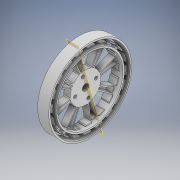
# Autodesk Inventor part: Kotač_v.3.0
Saved by Autodesk Inventor 2020 (Build 240168000, 168)
## iProperties
Created: 2020-10-18
Part Number: Kotač_v.3.0
Material: Generic
Document SubType Name: Modeling
Designer: Sičaja
Density: 1 g/cm^3
Appearance: Default
Author: Sičaja
Autodesk Inventor part; units mm, degrees
ref_plane "YZ Plane" through (0, 0, 0) normal (1, 0, 0) x (0, 1, 0)
ref_plane "XZ Plane" through (0, 0, 0) normal (0, 1, 0) x (-1, 0, 0)
ref_plane "XY Plane" through (0, 0, 0) normal (0, 0, 1) x (1, 0, 0)
sketch "Sketch1" plane through (0, 0, 0) normal (1, 0, 0) x (0, 1, 0)
  circle A0 centre (0, 0) radius 25
  dimension "d0" = 50
  constraints: 1 centre point, 1 coincident
  measures "d0" diameter of A0
extrude "Extrusion1" add sketch "Sketch1" along normal blind 7
sketch "Sketch3" plane through (7, 0, 0) normal (1, 0, 0) x (0, 0, -1)
  arc A0 (-3.1611, 20.2548) -> (-7.5525, 19.0581) centre (0, 0) ccw
  line L0 (-3.1611, 20.2548) -> (-1.4649, 9.3864)
  line L1 (-3.4999, 8.8318) -> (-7.5525, 19.0581)
  line L2 (-2.081, 9.2902) -> (-3.6795, 19.5329)
  arc A1 (-3.6795, 19.5329) -> (-6.7395, 18.699) centre (0, 0) ccw
  line L3 (-6.7395, 18.699) -> (-2.9203, 9.0615)
  circle A2 centre (0, 0) radius 9.5591
  line L4 (-17.9878, 8.4566) -> (-8.4724, 4.3425)
  line L5 (-8.7198, 3.7702) -> (-18.8165, 8.1357)
  arc A3 (-16.4137, 11.2101) -> (-17.9878, 8.4566) centre (0, 0) ccw
  arc A4 (-16.5575, 12.0871) -> (-18.8165, 8.1357) centre (0, 0) ccw
  line L6 (-16.5575, 12.0871) -> (-7.673, 5.6013)
  line L7 (-8.0406, 5.0977) -> (-16.4137, 11.2101)
  circle A5 centre (0, 0) radius 9.5591
  line L8 (-18.699, -6.7395) -> (-9.0615, -2.9203)
  line L9 (-8.8318, -3.4999) -> (-19.0581, -7.5525)
  arc A6 (-19.5329, -3.6795) -> (-18.699, -6.7395) centre (0, 0) ccw
  arc A7 (-20.2548, -3.1611) -> (-19.0581, -7.5525) centre (0, 0) ccw
  line L10 (-20.2548, -3.1611) -> (-9.3864, -1.4649)
  line L11 (-9.2902, -2.081) -> (-19.5329, -3.6795)
  circle A8 centre (0, 0) radius 9.5591
  line L12 (-8.4566, -17.9878) -> (-4.3425, -8.4724)
  line L13 (-3.7702, -8.7198) -> (-8.1357, -18.8165)
  arc A9 (-11.2101, -16.4137) -> (-8.4566, -17.9878) centre (0, 0) ccw
  arc A10 (-12.0871, -16.5575) -> (-8.1357, -18.8165) centre (0, 0) ccw
  line L14 (-12.0871, -16.5575) -> (-5.6013, -7.673)
  line L15 (-5.0977, -8.0406) -> (-11.2101, -16.4137)
  circle A11 centre (0, 0) radius 9.5591
  line L16 (6.7395, -18.699) -> (2.9203, -9.0615)
  line L17 (3.4999, -8.8318) -> (7.5525, -19.0581)
  arc A12 (3.6795, -19.5329) -> (6.7395, -18.699) centre (0, 0) ccw
  arc A13 (3.1611, -20.2548) -> (7.5525, -19.0581) centre (0, 0) ccw
  line L18 (3.1611, -20.2548) -> (1.4649, -9.3864)
  line L19 (2.081, -9.2902) -> (3.6795, -19.5329)
  circle A14 centre (0, 0) radius 9.5591
  line L20 (17.9878, -8.4566) -> (8.4724, -4.3425)
  line L21 (8.7198, -3.7702) -> (18.8165, -8.1357)
  arc A15 (16.4137, -11.2101) -> (17.9878, -8.4566) centre (0, 0) ccw
  arc A16 (16.5575, -12.0871) -> (18.8165, -8.1357) centre (0, 0) ccw
  line L22 (16.5575, -12.0871) -> (7.673, -5.6013)
  line L23 (8.0406, -5.0977) -> (16.4137, -11.2101)
  circle A17 centre (0, 0) radius 9.5591
  line L24 (18.699, 6.7395) -> (9.0615, 2.9203)
  line L25 (8.8318, 3.4999) -> (19.0581, 7.5525)
  arc A18 (19.5329, 3.6795) -> (18.699, 6.7395) centre (0, 0) ccw
  arc A19 (20.2548, 3.1611) -> (19.0581, 7.5525) centre (0, 0) ccw
  line L26 (20.2548, 3.1611) -> (9.3864, 1.4649)
  line L27 (9.2902, 2.081) -> (19.5329, 3.6795)
  circle A20 centre (0, 0) radius 9.5591
  line L28 (8.4566, 17.9878) -> (4.3425, 8.4724)
  line L29 (3.7702, 8.7198) -> (8.1357, 18.8165)
  arc A21 (11.2101, 16.4137) -> (8.4566, 17.9878) centre (0, 0) ccw
  arc A22 (12.0871, 16.5575) -> (8.1357, 18.8165) centre (0, 0) ccw
  line L30 (12.0871, 16.5575) -> (5.6013, 7.673)
  line L31 (5.0977, 8.0406) -> (11.2101, 16.4137)
  circle A23 centre (0, 0) radius 9.5591
  circle A24 centre (0, 0) radius 2 projected
  circle A25 centre (0, 0) radius 20.5
  circle A26 centre (0, 0) radius 9.5204
  point P0 (-8.5079, 4.3579)
  point P1 (-8.0719, 5.1206)
  point P2 (-9.4448, -1.474)
  point P3 (-8.7741, 3.7936)
  point P4 (-9.0975, -2.9345)
  point P5 (-9.3285, -2.0869)
  point P6 (-4.3579, -8.5079)
  point P7 (-5.1206, -8.0719)
  point P8 (-12.0871, -16.5575)
  point P9 (-5.6362, -7.7207)
  point P10 (-8.8867, -3.5217)
  point P11 (1.474, -9.4448)
  point P12 (-3.7936, -8.7741)
  point P13 (2.9345, -9.0975)
  point P14 (2.0869, -9.3285)
  point P15 (7.7207, -5.6362)
  point P16 (3.5217, -8.8867)
  point P17 (8.5079, -4.3579)
  point P18 (8.0719, -5.1206)
  point P19 (9.4448, 1.474)
  point P20 (8.7741, -3.7936)
  point P21 (9.0975, 2.9345)
  point P22 (9.3285, 2.0869)
  point P23 (19.0581, 7.5525)
  point P24 (5.6362, 7.7207)
  point P25 (8.8867, 3.5217)
  point P26 (4.3579, 8.5079)
  point P27 (5.1206, 8.0719)
  point P28 (-2.9345, 9.0975)
  point P29 (-2.0869, 9.3285)
  point P30 (-1.474, 9.4448)
  point P31 (3.7936, 8.7741)
  point P32 (-7.5525, 19.0581)
  point P33 (-16.5575, 12.0871)
  point P34 (-7.7207, 5.6362)
  point P35 (-3.5217, 8.8867)
  dimension "d15" = 41
  dimension "d18" = 360
  constraints: 64 end point, 32 point on circle, 24 centre point, 10 coincident, 2 coincident with centre, 142 other
  measures "d15" diameter of A0
extrude "Extrusion3" cut sketch "Sketch3" against normal blind 7 contours A25 L29 A2 L0 | L1 A2 L6 A25 | A2 L3 A1 L2 | A25 L25 A2 L30 | L5 A2 L10 A25 | L28 A21 L31 A2 | A2 L4 A3 L7 | A25 L21 A2 L26 | L9 A2 L14 A25 | L24 A18 L27 A2 | A2 L8 A6 L11 | L13 A2 L18 A25 | A25 L17 A2 L22 | A2 L12 A9 L15 | L20 A15 L23 A2 | A2 L16 A12 L19
sketch "Sketch4" plane through (7, 0, 0) normal (1, 0, 0) x (0, 0, -1)
  circle A0 centre (0, 0) radius 9.5
  circle A1 centre (0, 0) radius 7.8
  circle A2 centre (0, 0) radius 6.8
  circle A3 centre (0, 0) radius 2
  circle A4 centre (-1.787, 6.561) radius 1
  circle A5 centre (-6.561, -1.787) radius 1
  circle A6 centre (1.787, -6.561) radius 1
  circle A7 centre (6.561, 1.787) radius 1
  dimension "d24" = 13.6
  dimension "d22" = 19
  dimension "d23" = 15.6
  dimension "d25" = 4
  dimension "d26" = 2
  dimension "d29" = 360
  constraints: 7 centre point, 4 coincident, 12 other
  measures "d22" diameter of A0
  measures "d23" diameter of A1
  measures "d25" diameter of A3
  measures "d26" diameter of A4
extrude "Extrusion4" cut sketch "Sketch4" against normal blind 7 contours A7 A2 | A6 A2 | A4 A2 | A2 A7 | A5 A2 | A6 A2 | A4 A2 | A5 A2 | A3
sketch "Sketch5" plane through (7, 0, 0) normal (1, 0, 0) x (0, 0, -1)
  circle A0 centre (0, 0) radius 21.5
  circle A1 centre (0, 0) radius 25 projected
  circle A2 centre (0, 0) radius 23.5
  circle A3 centre (0, 0) radius 26
  dimension "d33" = 43
  dimension "d34" = 47
  dimension "d35" = 52
  constraints: 3 centre point, 3 coincident
  measures "d33" diameter of A0
  measures "d34" diameter of A2
  measures "d35" diameter of A3
extrude "Extrusion5" cut sketch "Sketch5" against normal blind 7 contours A1 | A2 | A3
ref_plane "Work Plane2" through (0, 0, 0) normal (0, -0.2629324, 0.9648142) x (-1, 0, 0)
sketch "Sketch8" plane through (0, 0, 0) normal (-1, 0, 0) x (0, 0, 1)
  circle A0 centre (0, 0) radius 2 projected
  line L0 (-0.9032, 19.8559) -> (-0.9315, 20.4788)
  line L1 (10.8505, 16.6535) -> (11.1909, 17.176)
  line L2 (5.2251, 19.1774) -> (5.6518, 20.7438)
  line L3 (2.0869, 9.3285) -> (3.6795, 19.5329) projected
  line L4 (3.1611, 20.2548) -> (1.474, 9.4448) projected
  line L5 (3.5217, 8.8867) -> (7.5525, 19.0581) projected
  line L6 (7.5525, 19.0581) -> (3.5217, 8.8867) projected
  line L7 (3.5217, 8.8867) -> (7.5525, 19.0581)
  line L8 (7.3228, 18.4784) -> (7.5525, 19.0581)
  arc A1 (10.8505, 16.6535) -> (7.3228, 18.4784) centre (0, 0) ccw
  arc A2 (3.0649, 19.6388) -> (-0.9032, 19.8559) centre (0, 0) ccw
  line L9 (3.0649, 19.6388) -> (3.1611, 20.2548)
  line L10 (3.0649, 19.6388) -> (3.1611, 20.2548)
  arc A3 (11.1909, 17.176) -> (7.5525, 19.0581) centre (0, 0) ccw
  arc A4 (3.1611, 20.2548) -> (-0.9315, 20.4788) centre (0, 0) ccw
  point P0 (14.1483, 21.715)
  constraints: 14 end point, 8 point on circle, 4 centre point, 1 coincident, 1 collinear
sketch "Sketch9" plane through (7, 0, 0) normal (1, 0, 0) x (0, 0, -1)
  circle A0 centre (0, 0) radius 20.5
  constraints: 1 centre point, 1 coincident
extrude "Extrusion7" cut sketch "Sketch9" against normal blind 3
extrude "Extrusion8" add sketch "Sketch8" against normal blind 5 contours L0 A4 L4 A2 | A1 L5 A3 L1
chamfer "Chamfer1" distance 0.5 angle 45 4 edges at (2.5, 19.8559, -0.9032) (5, 19.9468, 3.113) (2.5, 16.6535, 10.8505) (5, 18.7682, 7.4376)
pattern_circular "Circular Pattern1" count 8 over 360 about axis through (7, 0, 0) along (-1, 0, 0) of "Extrusion8", "Chamfer1"
chamfer "Chamfer2" distance 0.5 angle 45 15 edges at (2, 8.8867, 3.5217) (2, 9.4448, 1.474) (2, 7.7207, -5.6362) (2, 8.7741, -3.7936) (2, 3.5217, -8.8867) (2, -3.7936, -8.7741) (2, -5.6362, -7.7207) (2, -8.8867, -3.5217) (2, -9.4448, -1.474) (2, -7.7207, 5.6362) (2, -3.5217, 8.8867) (2, -8.7741, 3.7936) (2, -1.474, 9.4448) (2, 3.7936, 8.7741) (2, 5.6362, 7.7207)
fillet "Fillet1" radius 0.3 16 edges at (2, 16.4137, -11.2101) (2, 17.9878, -8.4566) (2, 6.7395, -18.699) (2, 19.5329, 3.6795) (2, 3.6795, -19.5329) (2, -8.4566, -17.9878) (2, -11.2101, -16.4137) (2, -18.699, -6.7395) (2, -19.5329, -3.6795) (2, -17.9878, 8.4566) (2, -16.4137, 11.2101) (2, -6.7395, 18.699) (2, -3.6795, 19.5329) (2, 8.4566, 17.9878) (2, 11.2101, 16.4137) (2, 18.699, 6.7395)
sketch "Sketch10" plane through (0, 0, 0) normal (0, -0.2629324, 0.9648142) x (-1, 0, 0)
  line L0 (-7, 21.5) -> (-7, -21.5) projected
  line L1 (1.4, 0) -> (-8.4, 0) projected
  line L2 (-7, 21.5) -> (-4.5, 21.5)
  line L3 (0, 21.5) -> (-7, 21.5) projected
  line L4 (-4.5, 21.5) -> (-4.5, 23)
  line L5 (-4.5, 23) -> (-2.5, 23)
  line L6 (-2.5, 23) -> (-2.5, 21.5)
  line L7 (0, 21.5) -> (-7, 21.5) projected
  line L8 (-2.5, 21.5) -> (-4.5, 21.5)
  point P0 (0, 0)
  dimension "d67" = 2.5
  dimension "d68" = 1.5
  dimension "d69" = 2
  constraints: 10 end point, 2 perpendicular, 2 point on line, 1 collinear, 1 vertical
  measures "d67" distance of L0.start L2.end
  measures "d68" distance of L2.end L4.end
  measures "d69" distance of L4.end L5.end
sketch "Sketch11" plane through (0, 0, 0) normal (0, -0.2629324, 0.9648142) x (-1, 0, 0)
  line L0 (-4.5, 22.4692) -> (-2.5, 22.4692) projected
  line L1 (-7, 21.5) -> (-7, -21.5) projected
  line L2 (-6.5, 23.4692) -> (-0.5, 23.4692)
  line L3 (-6.5, 23.4692) -> (-6.5, 22.9692)
  line L4 (-6.5, 22.9692) -> (-0.5, 22.9692)
  line L5 (-0.5, 22.9692) -> (-0.5, 23.4692)
  line L6 (1.4, 0) -> (-8.4, 0) projected
  point P0 (0, 0)
  dimension "d61" = 6
  dimension "d63" = 0.5
  constraints: 8 end point, 1 vertical
  measures "d61" distance of L2.start L2.end
  measures "d63" distance of L2.start L3.end
revolve "Revolution2" add sketch "Sketch10" angle 6 mid plane about axis through (4, 0, 0) along (1, 0, 0)
revolve "Revolution3" add sketch "Sketch11" angle 12 mid plane about axis through (4, 0, 0) along (1, 0, 0)
pattern_circular "Circular Pattern2" count 20 over 360 about axis through (4, 0, 0) along (1, 0, 0) of "Revolution2", "Revolution3"
sketch "Sketch12" plane through (0, 0, 0) normal (-1, 0, 0) x (0, 0, 1)
  circle A0 centre (0, 0) radius 2 projected
  circle A1 centre (0, 0) radius 25
  circle A2 centre (0, 0) radius 26
  dimension "d75" = 50
  dimension "d76" = 52
  constraints: 2 centre point, 2 coincident
  measures "d75" diameter of A1
  measures "d76" diameter of A2
extrude "Extrusion9" add sketch "Sketch12" against normal blind 7 contours A2
body "Solid1"
